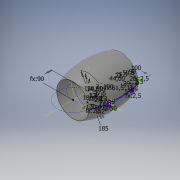
# Autodesk Inventor part: Form
Saved by Autodesk Inventor 2018.3 (Build 223284000, 284)
## iProperties
Created: 2018-07-22
Part Number: Form
Material: Generisch
Document SubType Name: Modeling
Designer: JochenAlt
Density: 1 g/cm^3
Appearance: Textur - grau
Author: JochenAlt
Autodesk Inventor part; units mm, degrees
ref_plane "YZ Plane" through (0, 0, 0) normal (1, 0, 0) x (0, 1, 0)
ref_plane "XY Plane" through (0, 0, 0) normal (0, 0, 1) x (1, 0, 0)
sketch "Skizze3" plane through (0, 0, 0) normal (0, 0, 1) x (1, 0, 0)
  line L0 (0, 294.302654) -> (0, -259.050443) construction
  line L1 (-139.25, 0) -> (205.5, 0) construction
  line L2 (102.5, 190) -> (100, 190)
  circle A0 centre (0, 0) radius 90 construction
  circle A1 centre (0, -90) radius 90 construction
  line L3 (93, -90) -> (95.5, -90)
  line L4 (93, -90) -> (128.84929, -11.665489) construction
  line L5 (128.84929, 127.691225) -> (100, 190) construction
  spline S0 degree 3 poles (93, -90) (128.84929, -11.665489) (128.84929, 127.691225) (100, 190) knots 1 1 1 1 2 2 2 2
  line L6 (102.5, 190) -> (130.84929, 128.771126) construction
  line L7 (130.84929, -12.758042) -> (95.5, -90) construction
  spline S1 degree 3 poles (102.5, 190) (130.84929, 128.771126) (130.84929, -12.758042) (95.5, -90) knots 1 1 1 1 2 2 2 2
  line L8 (153.75, 101.643763) -> (156.25, 101.643763) construction
  line L9 (153.75, 101.643763) -> (156.25, 101.643763) construction
  line L10 (130.84929, 128.771126) -> (130.84929, -12.758042) construction
  line L11 (128.84929, -11.665489) -> (128.84929, 127.691225) construction
  line L12 (62.519253, 64.740582) -> (105.240743, 108.97998) construction
  line L13 (62.519253, -25.259418) -> (105.240743, 18.97998) construction
  circle A2 centre (105.240743, 18.97998) radius 8.5 construction
  circle A3 centre (105.240743, 108.97998) radius 8.5 construction
  line L14 (93, -90) -> (90, -90) construction
  line L15 (113.705716, 18.209117) -> (118.685112, 17.755668) construction
  line L16 (113.700721, 109.803855) -> (118.677179, 110.288488) construction
  line L17 (111.750338, 139.045874) -> (114.703912, 139.571609) construction
  arc A4 (107.772562, 125.997321) -> (107.402341, 147.207293) centre (96.982465, 136.417196) ccw construction
  line L18 (107.402341, 147.207293) -> (52.408648, 200.314085) construction
  line L19 (107.772562, 125.997321) -> (64.474974, 81.161355) construction
  line L20 (102.5, 190) -> (91.930255, 212.828564) construction
  line L21 (91.930255, 212.828564) -> (92.5, 215) construction
  spline S2 degree 2 poles (102.5, 190) (91.930255, 212.828564) (92.5, 215) knots 1 1 1 2 2 2
  line L22 (100, 190) -> (89.430255, 212.828564) construction
  line L23 (89.430255, 212.828564) -> (90, 215) construction
  spline S3 degree 2 poles (100, 190) (89.430255, 212.828564) (90, 215) knots 1 1 1 2 2 2
  line L24 (92.5, 215) -> (90, 215)
  line L25 (100, 190) -> (100, 185)
  line L26 (100, 185) -> (98, 185)
  line L27 (98, 185) -> (98, 183)
  line L28 (98, 183) -> (102.994343, 183)
  line L29 (100, 190) -> (59.8, 190) construction
  line L30 (59.8, 190) -> (59.8, 185)
  line L31 (59.8, 185) -> (22, 172.5)
  arc A5 (49.958168, 183.745426) -> (59.8, 190) centre (42.463606, 206.408983) ccw
  line L32 (49.958168, 183.745426) -> (22, 174.5)
  line L33 (22, 174.5) -> (22, 172.5)
  line L34 (59.8, 185) -> (98, 185) construction
  line L35 (22, 174.5) -> (9.012369, 174.5)
  line L36 (9.012369, 174.5) -> (9.012369, 172.5)
  line L37 (9.012369, 172.5) -> (22, 172.5)
  point P0 (90, 149.814531)
  point P1 (22, 173.5)
  dimension "d13" = 180
  dimension "d108" = 17
  dimension "d7" = 190
  dimension "d11" = 2.5
  dimension "d14" = 90
  dimension "d15" = 100
  dimension "d18" = 2.5
  dimension "d19" = 2.5
  dimension "d105" = 2
  dimension "d106" = 61.5
  dimension "d107" = 44
  dimension "d110" = 3
  dimension "d111" = 5
  dimension "d112" = 5
  dimension "d119" = 10
  dimension "d120" = 15
  dimension "d121" = 29
  dimension "d122" = 3
  dimension "d127" = 2.5
  dimension "d128" = 90
  dimension "d129" = 25
  dimension "d137" = 5
  dimension "d149" = 2
  dimension "d181" = 2
  dimension "d183" = 59.8
  dimension "d184" = 22
  dimension "d185" = 15.5
  constraints: 52 end point, 10 horizontal, 9 point on circle, 8 parallel, 5 point on line, 4 perpendicular, 3 centre point, 3 equal length, 3 tangent, 3 vertical, 2 coincident, 2 line through centre, 1 collinear, 1 midpoint, 31 other
  measures "d7" distance between parallel lines of L1 L2
  measures "d11" distance of L2.start L2.end
  measures "d14" distance of A1.centre point (0, 0)
  measures "d15" distance from line of L0 L2.end
  measures "d18" distance of L3.end L3.start
  measures "d19" distance of L8.start L8.end
  measures "d105" distance between parallel lines of L10 L11
  measures "d106" distance of L12.start L12.end
  measures "d107" angle of L0 L12
  measures "d110" distance of L3.start L14.end
  measures "d111" distance of L15.start L15.end
  measures "d112" distance of L16.start L16.end
  measures "d119" distance from line of L19.start L12
  measures "d120" radius of A4
  measures "d121" distance from line of L18 point (105.241, 108.98)
  measures "d122" distance of L17.start L17.end
  measures "d127" distance of L21.end L23.end
  measures "d128" distance from line of L0 L23.end
  measures "d129" distance between parallel lines of L2 L24
  measures "d137" distance of L2.end L25.end
  measures "d149" distance of L26.end L27.end
  measures "d181" distance of L31.end L32.end
  measures "d183" distance between parallel lines of L30 L0
  measures "d184" distance between parallel lines of L0 L33
  measures "d185" distance between parallel lines of L35 L29
revolve "Umdrehung1" add sketch "Skizze3" angle 360 about axis through (0, 0, 0) along (0, -1, 0) contours S1 L3 S0 L2 | S0 L28 L27 L26 L25
sketch "Skizze6" plane through (0, 0, 0) normal (1, 0, 0) x (0, 1, 0)
  line L0 (-38, 0) -> (228, 0) construction
  line L1 (0, 126) -> (0, -126) construction
  line L2 (158.5, 25) -> (158.5, -25)
  line L3 (168.5, 25) -> (158.5, 25)
  line L4 (158.5, -25) -> (168.5, -25)
  line L5 (168.5, -25) -> (168.5, 25)
  line L6 (190, 100) -> (190, -100) projected
  point P0 (0, 0)
  point P1 (190, 0)
  dimension "d35" = 50
  dimension "d49" = 21.5
  dimension "d51" = 10
  constraints: 8 end point, 2 vertical, 1 horizontal, 1 parallel, 1 other
  measures "d35" distance of L2.start L2.end
  measures "d49" distance between parallel lines of L6 L5
  measures "d51" distance of L2.end L4.end
extrude "Extrusion4" add sketch "Skizze6" along normal up to next separate body
sketch "Skizze7" plane through (0, 0, 0) normal (0, 1, 0) x (-1, 0, 0)
  arc A0 (-91.711127, 12.054839) -> (-91.711127, -12.054839) centre (0, 0) ccw
  circle A1 centre (-77.5, 0) radius 7.6
  line L0 (-76.183742, -10.013864) -> (-91.711127, -12.054839)
  line L1 (-76.183742, 10.013864) -> (-91.711127, 12.054839)
  line L2 (-102.5, 0) -> (-122.959231, 0) construction
  arc A2 (-76.183742, -10.013864) -> (-76.183742, 10.013864) centre (-77.5, 0) ccw
  circle A3 centre (-77.5, 0) radius 6.6
  line L3 (-91.711127, -12.054839) -> (-127.5, -16.759056)
  line L4 (-91.711127, 12.054839) -> (-127.5, 16.759056)
  line L5 (-127.5, -16.759056) -> (-127.5, 16.759056)
  arc A4 (-49.9, 86.429335) -> (-49.9, -86.429335) centre (0, 0) ccw
  line L6 (-49.9, -86.429335) -> (-37.4, -64.7787)
  line L7 (-49.9, 86.429335) -> (-38.4, 66.510751)
  line L8 (-198.35277, 0) -> (138.058795, 0) construction
  circle A5 centre (0, 0) radius 85 construction
  circle A6 centre (0, 0) radius 100 construction
  circle A7 centre (-89.5, 0) radius 1.15
  circle A8 centre (-89.5, 0) radius 2.15 construction
  line L9 (-91.65, 1.241303) -> (-89.5, 2.482606)
  line L10 (-89.5, 2.482606) -> (-87.35, 1.241303)
  line L11 (-87.35, 1.241303) -> (-87.35, -1.241303)
  line L12 (-87.35, -1.241303) -> (-89.5, -2.482606)
  line L13 (-89.5, -2.482606) -> (-91.65, -1.241303)
  line L14 (-91.65, -1.241303) -> (-91.65, 1.241303)
  line L15 (0, -126) -> (0, 126) construction
  line L16 (-37.4, -64.7787) -> (0, 0)
  line L17 (-38.4, 66.510751) -> (0, 0)
  arc A9 (-48.9, 84.697284) -> (-48.9, -84.697284) centre (0, 0) ccw
  circle A10 centre (-43.264, 0) radius 12.7
  circle A11 centre (-43.264, 0) radius 8.5 construction
  circle A12 centre (-43.264, -8.5) radius 1.65
  circle A13 centre (-43.264, 8.5) radius 1.65
  circle A14 centre (-43.264, 0) radius 14.7
  circle A15 centre (-43.264, 0) radius 4
  line L18 (-43.264, 8.5) -> (-43.264, -8.5) construction
  line L19 (-44.732678, -16.817722) -> (-44.542871, -14.644265) construction
  line L20 (0, -25) -> (0, 25)
  line L21 (-77.901749, -33.501604) -> (-79.739055, -34.291736)
  line L22 (-77.901749, 33.501604) -> (-79.739055, 34.291736)
  arc A16 (-63.201737, 59.496054) -> (-79.739055, 34.291736) centre (0, 0) ccw
  arc A17 (-79.739055, -34.291736) -> (-63.201737, -59.496054) centre (0, 0) ccw
  line L23 (-61.745476, 58.125177) -> (-63.201737, 59.496054)
  line L24 (-61.745476, -58.125177) -> (-63.201737, -59.496054)
  arc A18 (-61.745476, 58.125177) -> (-77.901749, 33.501604) centre (0, 0) ccw
  arc A19 (-77.901749, -33.501604) -> (-61.745476, -58.125177) centre (0, 0) ccw
  arc A20 (-76.053419, -11.005335) -> (-76.053419, 11.005335) centre (-77.5, 0) ccw
  line L25 (-76.053419, -11.005335) -> (-83.940627, -12.042058)
  line L26 (-76.053419, 11.005335) -> (-83.940627, 12.042058)
  line L27 (-38.4, 66.510751) -> (-37.4, 64.7787)
  line L28 (-37.4, -64.7787) -> (-37.4, -64.7787)
  line L29 (-79.739055, 34.291736) -> (-77.901749, 33.501604)
  arc A21 (-46.65636, 70.811186) -> (-61.745476, 58.125177) centre (0, 0) ccw
  arc A22 (-61.745476, -58.125177) -> (-46.65636, -70.811186) centre (0, 0) ccw
  arc A23 (-77.901749, 33.501604) -> (-83.940627, 12.042058) centre (0, 0) ccw
  arc A24 (-83.940627, -12.042058) -> (-77.901749, -33.501604) centre (0, 0) ccw
  arc A25 (-57.9336, 0.9449) -> (-77.901749, 33.501604) centre (-90.987145, 3.07395) ccw
  arc A26 (-77.901749, -33.501604) -> (-57.9336, -0.9449) centre (-90.987145, -3.07395) ccw
  line L30 (-46.65636, -70.811186) -> (-11.033581, -9.110723)
  line L31 (-11.033581, 9.110723) -> (-46.65636, 70.811186)
  arc A27 (-61.745476, -58.125177) -> (-29.090638, -3.899463) centre (-142.046873, 27.177752) ccw
  arc A28 (-29.090638, 3.899463) -> (-61.745476, 58.125177) centre (-142.046873, -27.177752) ccw
  arc A29 (-11.033581, 9.110723) -> (-11.033581, -9.110723) centre (0, 0) ccw
  point P0 (-100, 0)
  point P1 (-95.5, 0)
  point P2 (-91.65, 0)
  point P3 (-28.564, 0)
  point P4 (-5.773503, 0)
  dimension "d132" = 4.3
  dimension "d32" = 185
  dimension "d40" = 15.2
  dimension "d53" = 1
  dimension "d56" = 50
  dimension "d101" = 170
  dimension "d116" = 0.2
  dimension "d130" = 2.3
  dimension "d140" = 2.5
  dimension "d141" = 120
  dimension "d142" = 77.5
  dimension "d148" = 12
  dimension "d150" = 25.4
  dimension "d151" = 17
  dimension "d152" = 3.3
  dimension "d153" = 2
  dimension "d154" = 8
  dimension "d159" = 34.236
  dimension "d187" = 20
  dimension "d188" = 1
  dimension "d189" = 2
  dimension "d192" = 15
  dimension "d194" = 2
  dimension "d195" = 5
  constraints: 56 end point, 47 point on circle, 28 centre point, 17 coincident, 16 tangent, 11 point on line, 5 equal length, 4 collinear, 3 midpoint, 3 parallel, 2 concentric, 2 horizontal alignment, 2 vertical, 1 equal radius, 1 line through centre, 22 other
  measures "d32" diameter of A0
  measures "d40" diameter of A1
  measures "d53" radial gap between concentric circles of A3 A1
  measures "d56" distance from line of L5 A1.centre
  measures "d101" diameter of A5
  measures "d130" diameter of A7
  measures "d140" radial gap between concentric circles of A2 A1
  measures "d141" angle of L17 L16
  measures "d142" distance of A2.centre L16.end
  measures "d148" distance of A7.centre A1.centre
  measures "d150" diameter of A10
  measures "d151" diameter of A11
  measures "d152" diameter of A12
  measures "d153" radial gap between concentric circles of A14 A10
  measures "d154" diameter of A15
  measures "d159" distance of A10.centre A1.centre
  measures "d187" angle of L21 L24
  measures "d188" radial gap between concentric circles of A20 A2
  measures "d189" radial gap between concentric circles of A18 A16
  measures "d192" radial gap between concentric circles of A24 A4
  measures "d194" radial gap between concentric circles of A4 A9
  measures "d195" distance between parallel lines of L30 L16
extrude "Extrusion5" cut sketch "Skizze7" along normal through all both and the other way through all contours L1 A2 L0 A0 | A0 L3 A9 L4 | A9 L3 A4 L4 | A4 L3 L5 L4 | L9 L10 L11 L12 L13 L14 keep common part bodies 2
extrude "Extrusion8" add sketch "Skizze7" along normal blind 7 from surface at 158.5 contours A1 bodies 2
extrude "Extrusion9" add sketch "Skizze7" along normal blind 1 from surface at 158.5 contours A1 bodies 2
extrude "Extrusion16" cut sketch "Skizze7" along normal blind 5 from surface at 158.5 contours A7 | L9 L10 L11 L12 L13 L14 bodies 1 2
pattern_circular "Runde Anordnung2" count 3 over 360 about axis through (0, -10, 0) along (0, 1, 0) bodies 2
combine bodies "Kombinieren2" operation type add bodies to combine 2 1
extrude "Extrusion10" add sketch "Skizze7" against normal blind 1 from surface at 190 separate body contours L1 A2 L0 A0 | L4 A9 L7 L17 L16 L6 L3 L0 A2 L1 | A0 L3 A9 L4 | A9 L3 A4 L4 | L4 A4 L7 A9 | A9 L6 A4 L3 | A1 | L9 L10 L11 L12 L13 L14 | A18 L22 A16 L23 | L24 A17 L21 A19
extrude "Extrusion11" add sketch "Skizze7" against normal blind 4 from surface at 189 contours L1 A2 L0 A0 | L4 A9 L7 L17 L16 L6 L3 L0 A2 L1 | A0 L3 A9 L4 | A9 L3 A4 L4 | L4 A4 L7 A9 | A9 L6 A4 L3 | L9 L10 L11 L12 L13 L14 | A18 L22 A16 L23 | L24 A17 L21 A19 bodies 3
extrude "Extrusion17" cut sketch "Skizze7" against normal blind 2 from surface at 190 contours A9 L3 A4 L4 | L4 A4 L7 A9 | A9 L6 A4 L3 bodies 3
pattern_circular "Runde Anordnung3" count 3 over 360 about axis through (0, -10, 0) along (0, 1, 0) of "Extrusion10", "Extrusion11", "Extrusion17" bodies 3
ref_plane "MotorGear" through (77.5, 174.5, 0) normal (0, 1, 0) x (1, 0, 0)
extrude "Extrusion18" add sketch "Skizze7" against normal blind 2 from surface at 174.5 contours A10 | A14 | A14 A25 A18 A28 | A27 A19 A26 A14 | A18 L22 A16 L23 | L24 A17 L21 A19 bodies 3
extrude "Extrusion19" add sketch "Skizze7" against normal blind 5 from surface at 174.5 contours A14 bodies 3
extrude "Extrusion21" add sketch "Skizze7" along normal up to surface (10.5 mm away) from surface at 174.5 contours A18 L22 A16 L23 | L24 A17 L21 A19 bodies 3
fillet "Rundung3" radius 10 2 edges at (70.9008, 174.5, 46.5201) (70.9008, 174.5, -46.5201)
fillet "Rundung4" radius 12 2 edges at (72.5729, 172.5, -47.6173) (72.5729, 172.5, 47.6173)
sketch "Schnnitt" plane through (0, 50, 0) normal (0, 1, 0) x (-1, 0, 0)
  line L0 (0, 0) -> (161.461158, 0)
  line L1 (0, 0) -> (-80.730579, 139.829464)
  line L2 (0, 0) -> (-80.730579, -139.829464)
  circle A0 centre (0, 0) radius 161.461158
  line L3 (226.045621, 0) -> (-226.045621, 0) construction
  line L4 (0, -226.045621) -> (0, 226.045621) construction
  dimension "d123" = 120
  constraints: 6 end point, 3 point on circle, 1 centre point, 1 coincident, 1 horizontal, 1 other
  measures "d123" angle of L2 L1
equation "\"d14\" = 0.5 * d13"
equation "\"d18\" = d17"
equation "\"d16\" = d11"
equation "\"d17\" = d16"
